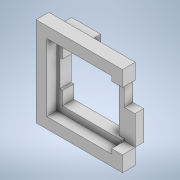
# Autodesk Inventor part: Camera Mod
Saved by Autodesk Inventor 2020 (Build 240168000, 168)
## iProperties
Created: 2021-04-05
Part Number: Camera Mod
Material: Generic
Document SubType Name: Modeling
Designer: 19166
Density: 1 g/cm^3
Appearance: Default
Author: 19166
Autodesk Inventor part; units mm, degrees
ref_plane "YZ Plane" through (0, 0, 0) normal (1, 0, 0) x (0, 1, 0)
ref_plane "XZ Plane" through (0, 0, 0) normal (0, 1, 0) x (-1, 0, 0)
ref_plane "XY Plane" through (0, 0, 0) normal (0, 0, 1) x (1, 0, 0)
sketch "Sketch1" plane through (0, 0, 0) normal (0, 0, 1) x (1, 0, 0)
  line L0 (0, 0) -> (0, 24) construction
  line L1 (0, 24) -> (1.113, 24) construction
  line L2 (1.113, 24) -> (1.113, 28) construction
  line L3 (1.113, 28) -> (12.113, 28) construction
  line L4 (12.113, 28) -> (12.113, 24) construction
  line L5 (12.113, 24) -> (24, 24) construction
  line L6 (24, 24) -> (24, 12.1) construction
  line L7 (24, 12.1) -> (28, 12.1) construction
  line L8 (28, 12.1) -> (28, 1.1) construction
  line L9 (28, 1.1) -> (24, 1.1) construction
  line L10 (24, 1.1) -> (24, 0) construction
  line L11 (24, 0) -> (0, 0) construction
  line L12 (12.013, 27.9) -> (1.213, 27.9)
  line L13 (1.213, 27.9) -> (1.213, 23.9)
  line L14 (1.213, 23.9) -> (0.1, 23.9)
  line L15 (0.1, 23.9) -> (0.1, 0.1)
  line L16 (0.1, 0.1) -> (23.9, 0.1)
  line L17 (23.9, 0.1) -> (23.9, 1.2)
  line L18 (23.9, 1.2) -> (27.9, 1.2)
  line L19 (27.9, 1.2) -> (27.9, 12)
  line L20 (27.9, 12) -> (23.9, 12)
  line L21 (23.9, 12) -> (23.9, 23.9)
  line L22 (23.9, 23.9) -> (12.013, 23.9)
  line L23 (12.013, 23.9) -> (12.013, 27.9)
  circle A0 centre (-1.945, 26.005) radius 1.548
  circle A1 centre (26.025, 26.005) radius 1.548
  circle A2 centre (-2.025, -2.005) radius 1.548
  circle A3 centre (26.025, -2.005) radius 1.548
  line L24 (0.1, 23.9) -> (23.9, 0.1) construction
  line L25 (23.9, 23.9) -> (0.1, 0.1) construction
  line L26 (-1.945, 26.005) -> (26.025, -2.005) construction
  line L27 (-2.025, -2.005) -> (26.025, 26.005) construction
  line L28 (2, 22) -> (22, 22)
  line L29 (22, 22) -> (22, 2)
  line L30 (22, 2) -> (2, 2)
  line L31 (2, 2) -> (2, 22) construction
  line L32 (2, 17) -> (1.05, 17)
  line L33 (1.05, 17) -> (1.05, 7)
  line L34 (1.05, 7) -> (2, 7)
  line L35 (2, 17) -> (2, 22)
  line L36 (2, 7) -> (2, 2)
  point P0 (12, 12)
  point P1 (1.05, 12)
  point P2 (12, 12)
  dimension "d0" = 24
  dimension "d1" = 1.113
  dimension "d2" = 4
  dimension "d3" = 11
  dimension "d4" = 11.887
  dimension "d5" = 11.9
  dimension "d6" = 4
  dimension "d7" = 11
  dimension "d8" = 1.1
  dimension "d9" = 0.1
  dimension "d10" = 3.096
  dimension "d11" = 27.97
  dimension "d12" = 28.01
  dimension "d15" = 20
  dimension "d16" = 0.95
  dimension "d17" = 10
  constraints: 74 end point, 17 perpendicular, 8 point on line, 6 horizontal, 4 centre point, 4 midpoint, 3 equal radius, 3 horizontal alignment, 3 vertical, 1 collinear, 1 vertical alignment, 11 other
  measures "d0" distance of L0.start L0.end
  measures "d1" distance of L0.end L1.end
  measures "d2" distance of L1.end L2.end
  measures "d3" distance of L2.end L3.end
  measures "d4" distance of L4.end L5.end
  measures "d5" distance of L5.end L6.end
  measures "d6" distance of L6.end L7.end
  measures "d7" distance of L7.end L8.end
  measures "d8" distance of L9.end L10.end
  measures "d9" distance between parallel lines of L3 L12
  measures "d10" diameter of A0
  measures "d11" distance of L27.end L26.start
  measures "d12" vertical distance of L27.start L26.start
  measures "d15" distance between parallel lines of L30 L28
  measures "d16" distance between parallel lines of L33 L15
  measures "d17" distance between parallel lines of L34 L32
extrude "Extrusion1" add sketch "Sketch1" along normal blind 3.2 contours L23 L22 L21 L20 L19 L18 L17 L16 L15 L14 L13 L12
sketch "Sketch2" plane through (0, 0, 3.2) normal (0, 0, 1) x (1, 0, 0)
  line L0 (0, 24.535) -> (24, 24.535)
  line L1 (24, 24.535) -> (24, -0.535) construction
  line L2 (24, -0.535) -> (0, -0.535)
  line L3 (0, -0.535) -> (0, 24.535)
  line L4 (22, 22) -> (22, 2) projected
  line L5 (1.3564, 23.1456) -> (22, 2) construction
  line L6 (22, 22) -> (2.0347, 2) construction
  line L7 (2, 22) -> (22, 22) projected
  line L8 (28, 28.535) -> (-4, 28.535)
  line L9 (-4, 28.535) -> (-4, -4.535)
  line L10 (-4, -4.535) -> (28, -4.535)
  line L11 (28, -4.535) -> (28, 28.535)
  line L12 (24, 1.2) -> (28, 1.2)
  line L13 (24, 22.8) -> (28, 22.8)
  line L14 (24, 24.535) -> (24, 22.8)
  line L15 (24, -0.535) -> (24, 1.2)
  line L16 (23.9, 0.1) -> (23.9, 1.2) projected
  point P0 (0, 0)
  point P1 (12, 24.535)
  point P2 (12, 22)
  point P3 (24, 12)
  point P4 (22, 12)
  dimension "d18" = 25.07
  dimension "d19" = 24
  dimension "d20" = 4
  dimension "d21" = 1.735
  dimension "d22" = 1.735
  constraints: 28 end point, 5 parallel, 5 point on line, 4 midpoint, 3 perpendicular, 2 horizontal, 1 collinear, 1 horizontal alignment, 1 vertical alignment, 3 other
  measures "d18" distance between parallel lines of L2 L0
  measures "d19" distance of L0.start L0.end
  measures "d20" distance between parallel lines of L0 L8
  measures "d21" distance between parallel lines of L13 L0
  measures "d22" distance between parallel lines of L12 L2
extrude "Extrusion2" add sketch "Sketch2" along normal blind 4.75 contours L3 L2 L15 L12 L11 L10 L9 L8 L13 L14 L0
sketch "Sketch3" plane through (0, 0, 3.2) normal (0, 0, 1) x (1, 0, 0)
  line L0 (28, 1.2) -> (24, 1.2) projected
  line L1 (24, 1.2) -> (24, -0.535) projected
  line L2 (24, -0.535) -> (0, -0.535) projected
  line L3 (0, -0.535) -> (0, 24.535) projected
  line L4 (0, 24.535) -> (24, 24.535) projected
  line L5 (24, 24.535) -> (24, 22.8) projected
  line L6 (24, 22.8) -> (28, 22.8) projected
  line L7 (28, 22.8) -> (28, 28.535) projected
  line L8 (28, 28.535) -> (-4, 28.535) projected
  line L9 (-4, 28.535) -> (-4, -4.535) projected
  line L10 (-4, -4.535) -> (28, -4.535) projected
  line L11 (28, -4.535) -> (28, 1.2) projected
  line L12 (12.013, 24.535) -> (1.213, 24.535) projected
  line L13 (1.213, 24.535) -> (1.213, 23.9) projected
  line L14 (1.213, 23.9) -> (0.1, 23.9) projected
  line L15 (0.1, 23.9) -> (0.1, 0.1) projected
  line L16 (0.1, 0.1) -> (23.9, 0.1) projected
  line L17 (23.9, 0.1) -> (23.9, 1.2) projected
  line L18 (23.9, 1.2) -> (24, 1.2) projected
  line L19 (24, 1.2) -> (27.9, 1.2) projected
  line L20 (27.9, 1.2) -> (27.9, 12) projected
  line L21 (27.9, 12) -> (23.9, 12) projected
  line L22 (23.9, 12) -> (23.9, 23.9) projected
  line L23 (23.9, 23.9) -> (12.013, 23.9) projected
  line L24 (12.013, 23.9) -> (12.013, 24.535) projected
  line L25 (22, 22) -> (22, 2) projected
  line L26 (22, 2) -> (2, 2) projected
  line L27 (2, 2) -> (2, 7) projected
  line L28 (2, 7) -> (1.05, 7) projected
  line L29 (1.05, 7) -> (1.05, 17) projected
  line L30 (1.05, 17) -> (2, 17) projected
  line L31 (2, 17) -> (2, 22) projected
  line L32 (2, 22) -> (22, 22) projected
  line L33 (0, 24.535) -> (1.213, 24.535) projected
  line L34 (0, 24.535) -> (24, 24.535)
  line L35 (24, 24.535) -> (24, 22.8) projected
  line L36 (2, 22) -> (22, 22) projected
  line L37 (12.013, 24.535) -> (24, 24.535) projected
  line L38 (24, 24.535) -> (24, 22)
  line L39 (2, 17) -> (2, 22) projected
  line L40 (24, 22) -> (2, 22)
  line L41 (2, 22) -> (2, 17)
  line L42 (1.05, 7) -> (1.05, 17) projected
  line L43 (2, 17) -> (1.05, 17)
  line L44 (1.05, 17) -> (1.05, 7)
  line L45 (2, 2) -> (2, 7) projected
  line L46 (1.05, 7) -> (2, 7)
  line L47 (2, 7) -> (2, 2)
  line L48 (2, 2) -> (24, 2)
  line L49 (24, 2) -> (24, 1.2)
  line L50 (24, 1.2) -> (24, -0.535) projected
  line L51 (24, 1.2) -> (24, -0.535)
  line L52 (24, -0.535) -> (0, -0.535)
  line L53 (0, -0.535) -> (0, 24.535) projected
  line L54 (0, 24.535) -> (0, -0.535)
  line L55 (24, -0.535) -> (0, -0.535) projected
  line L56 (0, -0.535) -> (24, -0.535)
  line L57 (24, -0.535) -> (24, 2)
  point P0 (0, 0)
  point P1 (23.9, 22)
  constraints: 30 end point, 7 collinear, 6 perpendicular, 1 horizontal, 1 point on line, 1 vertical
extrude "Extrusion3" add sketch "Sketch3" along normal blind 1 contours L1 L2 L3 L4 L13 L14 L15 L16 L17 L18 | L18 L17 L16 L15 L14 L13 L4 L24 L23 L22 L40 L32 L31 L30 L29 L28 L27 L26 L48 L49 | L22 L23 L24 L4 L5 L38 L40
body "Solid1"
